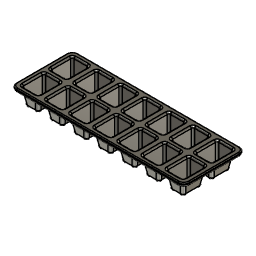
day5-icecube_tray (Autodesk Fusion 360 design; units mm, degrees)
part number: 2025-06-20-20-04-59-692
part number: 2025-06-20-20-23-34-543
Autodesk Fusion 360 part; units mm, degrees
sketch "Sketch1" plane through (0, 0, 0) normal (0, 0, 1) x (1, 0, 0) in component "tray"
  line L0 (0, 0) -> (300, 0)
  line L1 (300, 0) -> (300, 104)
  line L2 (300, 104) -> (0, 104)
  line L3 (0, 104) -> (0, 0)
  dimension "d1" = 300
  dimension "d2" = 104
  constraint horizontal L0
  constraint vertical L1
  constraint horizontal L2
  constraint vertical L3
  constraint coincident L0.start L3.end
  measures "d1" distance of L0.start L0.end
  measures "d2" distance of L0.start L2.end
extrude "Extrude1" add sketch "Sketch1" along normal blind 50 in component "tray"
sketch "Sketch2" plane through (0, 0, 50) normal (0, 0, 1) x (-1, 0, 0) in component "tray"
  line L0 (0, -104) -> (0, 0)
  line L1 (0, 0) -> (-300, 0)
  line L2 (-300, 0) -> (-300, -104)
  line L3 (-300, -104) -> (0, -104)
  line L4 (-7, -97) -> (-37, -97)
  line L5 (-37, -97) -> (-37, -57)
  line L6 (-37, -57) -> (-7, -57)
  line L7 (-7, -57) -> (-7, -97)
  dimension "d5" = 30
  dimension "d6" = 40
  dimension "d7" = 7
  dimension "d8" = 7
  constraint horizontal L4
  constraint vertical L5
  constraint horizontal L6
  constraint vertical L7
  measures "d5" distance of L4.start L4.end
  measures "d6" distance of L4.start L6.end
  measures "d7" distance of L0 L7
  measures "d8" distance of L3 L4
extrude "Extrude2" cut sketch "Sketch2" against normal blind 30 draft -10 contours L4 L5 L6 L7 in component "tray"
fillet "Fillet1" radius 3 4 edges at (7, 77, 50) (22, 57, 50) (37, 77, 50) (22, 97, 50) 4 faces at (8.7633, 72.0966, 40) (18.7633, 95.2367, 40) (25.2367, 58.7633, 40) (35.2367, 81.9034, 40) in component "tray"
pattern_linear "R-Pattern1" count 2 spacing 50 along (0, -1, 0) count 7 spacing 42.5 along (1, 0, 0) of "Extrude2", "Fillet1" in component "tray"
shell "Shell1" thickness 2 removed faces 5 at (200, 104, 16.6667) at (300, 34.6667, 16.6667) at (100, 0, 16.6667) at (0, 69.3333, 16.6667) at (100, 69.3333, 0) in component "tray"
fillet "Fillet2" radius 8 4 edges at (300, 0, 49) (0, 0, 49) (0, 104, 49) (300, 104, 49) in component "tray"
ref_plane "WorkPlane1" through (150, 52, 49) normal (0, 1, 0) x (-1, 0, 0) in component "tray"
sketch "Sketch3" plane through (0, 52, 0) normal (0, 1, 0) x (1, 0, 0) in component "tray"
  line L0 (0, -50) -> (0, -45)
  line L1 (0, -45) -> (-5, -45)
  line L2 (-5, -45) -> (-5, -47)
  line L3 (-5, -47) -> (-2, -47)
  line L4 (-2, -47) -> (-2, -50)
  line L5 (-2, -50) -> (0, -50)
  point P0 (0, -50)
  dimension "d20" = 2
  dimension "d21" = 3
  dimension "d22" = 5
  constraint vertical L0
  constraint perpendicular L0 L1
  constraint perpendicular L1 L2
  constraint perpendicular L2 L3
  constraint perpendicular L3 L4
  constraint perpendicular L0 L5
  constraint equal L2 L5
  constraint coincident P0 L0.start
  measures "d20" distance of P0 L4.end
  measures "d21" distance of L3.end L4.end
  measures "d22" distance of L0.end L1.end
sweep "Sweep1" add profiles "Sketch3" along 8 edges at (297.6569, 2.3431, 50) (300, 52, 50) (297.6569, 101.6569, 50) (150, 104, 50) (2.3431, 101.6569, 50) (0, 52, 50) (2.3431, 2.3431, 50) (150, 0, 50) section 1 in component "tray"
fillet "Fillet3" radius 1.55 32 edges at (302, 52, 50) (299.0711, 103.0711, 50) (150, 106, 50) (0.9289, 103.0711, 50) (-2, 52, 50) (0.9289, 0.9289, 50) (150, -2, 50) (299.0711, 0.9289, 50) (305, 52, 47) (301.1924, 105.1924, 47) (150, 109, 47) (-1.1924, 105.1924, 47) (-5, 52, 47) (-1.1924, -1.1924, 47) (150, -5, 47) (301.1924, -1.1924, 47) (302, 52, 47) (299.0711, 103.0711, 47) (150, 106, 47) (0.9289, 103.0711, 47) (-2, 52, 47) (0.9289, 0.9289, 47) (150, -2, 47) (299.0711, 0.9289, 47) (305, 52, 45) (301.1924, 105.1924, 45) (150, 109, 45) (-1.1924, 105.1924, 45) (-5, 52, 45) (-1.1924, -1.1924, 45) (150, -5, 45) (301.1924, -1.1924, 45) in component "tray"
component "tray" placed x (1, 0, 0) y (0, 1, 0) z (0, 0, 1) at (0, 0, 0)
